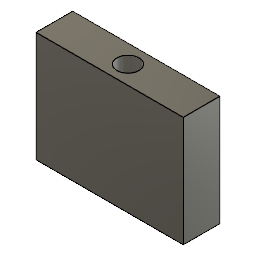
Endstop Y (Autodesk Fusion 360 design; units mm, degrees)
Autodesk Fusion 360 part; units mm, degrees
sketch "Skizze1" plane through (0, 0, 0) normal (0, 1, 0) x (1, 0, 0)
  line L0 (0, 0) -> (20, 0)
  line L1 (20, 0) -> (20, -5)
  line L2 (20, -5) -> (0, -5)
  line L3 (0, -5) -> (0, 0)
  constraint coincident L0.start L3.end
  constraint horizontal L0
  constraint perpendicular L0 L1
  constraint perpendicular L1 L2
  constraint perpendicular L0 L3
extrude "Extrusion1" add sketch "Skizze1" along normal blind 15
sketch "Skizze2" plane through (0, 15, 0) normal (0, 1, 0) x (-1, 0, 0)
  line L0 (0, 5) -> (-20, 5)
  line L1 (-20, 5) -> (-20, 0)
  line L2 (-20, 0) -> (0, 0)
  line L3 (0, 0) -> (0, 5)
  circle A0 centre (-10, 2.5) radius 1.5
  dimension "d3" = 3
  measures "d3" diameter of A0
extrude "Extrusion2" cut sketch "Skizze2" against normal blind 23 contours A0
